Autodesk Fusion 360 part; units mm, degrees
note: some values were not read from the file. Chosen so that the rebuilt part matches the saved one: which bodies a step acts on; which face or edge a step refers to. Set by a fixed rule: which sketch regions a step uses.
(part 2 of 2)
sketch "Sketch2 (7)" plane through (0, 0, 0) normal (0.707107, 0, -0.707107) x (-0.707107, 0, -0.707107) in component "left (1) (1)"
  line L0 (273.05, 19.05) -> (228.6, 19.05)
  line L1 (228.6, 19.05) -> (228.6, 0)
  line L2 (228.6, 0) -> (273.05, 0)
  line L3 (273.05, 0) -> (273.05, 19.05)
  line L4 (234.95, 12.7) -> (266.7, 12.7)
  line L5 (266.7, 12.7) -> (266.7, 6.35)
  line L6 (266.7, 6.35) -> (234.95, 6.35)
  line L7 (234.95, 6.35) -> (234.95, 12.7)
  line L8 (243.84, 12.7) -> (243.84, 19.05) construction
  line L9 (261.9443, 6.35) -> (261.9443, 0) construction
  line L10 (266.7, 9.6711) -> (273.05, 9.6711) construction
  line L11 (234.95, 7.62) -> (228.6, 7.62) construction
  dimension "d230_1" = 6.35
  dimension "d231_1" = 6.35
  constraint horizontal L4
  constraint vertical L5
  constraint horizontal L6
  constraint vertical L7
  constraint coincident L4 L8.start
  constraint coincident L0 L8.end
  constraint perpendicular L0 L8
  constraint coincident L6 L9.start
  constraint perpendicular L6 L9
  constraint coincident L5 L10.start
  constraint coincident L3 L10.end
  constraint perpendicular L3 L10
  constraint coincident L7 L11.start
  constraint coincident L1 L11.end
  constraint perpendicular L1 L11
  constraint equal L10 L11
  constraint equal L8 L9
  constraint coincident L2 L9.end
  measures "d230_1" distance of L11.start L11.end
  measures "d231_1" distance of L8.start L8.end
extrude "Extrude2''''''''" cut sketch "Sketch2 (7)" against normal blind 12.7 contours L4 L5 L6 L7 bodies 23 in component "left (1) (1)"
sketch "Sketch1 (15)" plane through (0, 0, 0) normal (0.707107, 0, 0.707107) x (0.707107, 0, -0.707107) in component "front (1) (1)"
  line L0 (273.05, 0) -> (273.05, 19.05)
  line L1 (273.05, 19.05) -> (228.6, 19.05)
  line L2 (228.6, 19.05) -> (228.6, 0)
  line L3 (228.6, 0) -> (273.05, 0)
  line L4 (234.95, 12.7) -> (266.7, 12.7)
  line L5 (266.7, 12.7) -> (266.7, 6.35)
  line L6 (266.7, 6.35) -> (234.95, 6.35)
  line L7 (234.95, 6.35) -> (234.95, 12.7)
  line L8 (234.95, 11.43) -> (228.6, 11.43) construction
  line L9 (241.3, 12.7) -> (241.3, 19.05) construction
  line L10 (245.7528, 6.35) -> (245.7528, 0) construction
  line L11 (266.7, 9.525) -> (273.05, 9.525) construction
  dimension "d234_1" = 6.35
  dimension "d235_1" = 6.35
  dimension "d242_1" = 6.35
  dimension "d243_1" = 31.75
  constraint horizontal L4
  constraint vertical L5
  constraint horizontal L6
  constraint vertical L7
  constraint coincident L7 L8.start
  constraint coincident L2 L8.end
  constraint perpendicular L2 L8
  constraint coincident L4 L9.start
  constraint coincident L1 L9.end
  constraint perpendicular L1 L9
  constraint coincident L6 L10.start
  constraint coincident L3 L10.end
  constraint perpendicular L3 L10
  constraint coincident L5 L11.start
  constraint perpendicular L5 L11
  constraint equal L9 L10
  constraint equal L8 L11
  constraint midpoint L0 L11.end
  measures "d234_1" distance of L11.start L11.end
  measures "d235_1" distance of L10.start L10.end
  measures "d242_1" distance of L4.start L6.end
  measures "d243_1" distance of L4.start L4.end
extrude "Extrude1''''''''''''''" cut sketch "Sketch1 (15)" against normal blind 12.7 contours L4 L5 L6 L7 bodies 21 in component "front (1) (1)"
sketch "Sketch2 (8)" plane through (0, 0, 0) normal (-0.707107, 0, 0.707107) x (0.707107, 0, 0.707107) in component "front (1) (1)"
  line L0 (-228.6, 19.05) -> (-273.05, 19.05)
  line L1 (-273.05, 19.05) -> (-273.05, 0)
  line L2 (-273.05, 0) -> (-228.6, 0)
  line L3 (-228.6, 0) -> (-228.6, 19.05)
  line L4 (-266.7, 12.7) -> (-234.95, 12.7)
  line L5 (-234.95, 12.7) -> (-234.95, 6.35)
  line L6 (-234.95, 6.35) -> (-266.7, 6.35)
  line L7 (-266.7, 6.35) -> (-266.7, 12.7)
  line L8 (-241.3, 12.7) -> (-241.3, 19.05) construction
  line L9 (-234.95, 10.16) -> (-228.6, 10.16) construction
  line L10 (-266.7, 9.525) -> (-273.05, 9.525) construction
  line L11 (-256.54, 6.35) -> (-256.54, 0) construction
  dimension "d238_1" = 6.35
  dimension "d239_1" = 6.35
  dimension "d244_1" = 6.35
  dimension "d245_1" = 31.75
  constraint horizontal L4
  constraint vertical L5
  constraint horizontal L6
  constraint vertical L7
  constraint coincident L4 L8.start
  constraint coincident L0 L8.end
  constraint perpendicular L0 L8
  constraint coincident L5 L9.start
  constraint coincident L3 L9.end
  constraint perpendicular L3 L9
  constraint midpoint L7 L10.start
  constraint coincident L1 L10.end
  constraint perpendicular L1 L10
  constraint coincident L6 L11.start
  constraint coincident L2 L11.end
  constraint perpendicular L2 L11
  constraint equal L8 L11
  constraint equal L9 L10
  measures "d238_1" distance of L10.start L10.end
  measures "d239_1" distance of L11.start L11.end
  measures "d244_1" distance of L4.end L5.end
  measures "d245_1" distance of L5.end L6.end
extrude "Extrude2'''''''''" cut sketch "Sketch2 (8)" against normal blind 12.7 contours L4 L5 L6 L7 bodies 21 in component "front (1) (1)"
sketch "Sketch1 (16)" plane through (0, 6.35, 0) normal (0, 1, 0) x (-1, 0, 0) in component "LargeConnector (1)"
  line L0 (-207.5446, 207.5446) -> (-166.1347, 166.1347)
  line L1 (-166.1347, 166.1347) -> (-157.1545, 175.115)
  line L2 (-157.1545, 175.115) -> (-198.5644, 216.5249)
  line L3 (-198.5644, 216.5249) -> (-207.5446, 207.5446)
  line L4 (-219.9225, 194.7967) -> (-178.7929, 153.6671)
  line L5 (-178.7929, 153.6671) -> (-196.3942, 136.0658)
  line L6 (-196.3942, 136.0658) -> (-237.5238, 177.1954)
  line L7 (-237.5238, 177.1954) -> (-219.9225, 194.7967)
  dimension "d267_1" = 12.7
  dimension "d268_1" = 12.7
  dimension "d269_1" = 58.5624
  dimension "d270_1" = 58.166
  dimension "d271_1" = 24.892
  constraint parallel L1 L5
  constraint parallel L3 L7
  constraint parallel L0 L6
  constraint parallel L2 L4
  measures "d267_1" distance of L0.start L2.end
  measures "d268_1" distance of L0.end L1.end
  measures "d269_1" distance of L1.end L2.end
  measures "d270_1" distance of L4.start L4.end
  measures "d271_1" distance of L4.end L5.end
extrude "Extrude1'''''''''''''''" add sketch "Sketch1 (16)" along normal blind 5.842 separate body contours L4 L5 L6 L7 makes body 28 in component "LargeConnector (1)"
fillet "Fillet1''" radius 1.27 1 edges at (237.5238, 9.271, 177.1954) on bodies 28 in component "LargeConnector (1)"
fillet "Fillet2''" radius 1.27 3 edges at (228.2741, 12.192, 186.4451) (236.9977, 12.192, 177.1954) (216.51, 12.192, 156.1816) on bodies 28 in component "LargeConnector (1)"
fillet "Fillet3''" radius 1.27 3 edges at (216.51, 6.35, 156.1816) (236.9977, 6.35, 177.1954) (228.2741, 6.35, 186.4451) on bodies 28 in component "LargeConnector (1)"
fillet "Fillet4''" radius 1.27 5 edges at (198.9087, 12.192, 173.7829) (219.6595, 11.82, 194.5337) (219.9225, 9.271, 194.7967) (219.6595, 6.722, 194.5337) (198.9087, 6.35, 173.7829) on bodies 28 in component "LargeConnector (1)"
fillet "Fillet5''" radius 1.27 8 edges at (196.3942, 9.271, 136.0658) (196.1312, 11.82, 136.3289) (187.5936, 12.192, 144.8665) (179.0559, 11.82, 153.4041) (178.7929, 9.271, 153.6671) (179.0559, 6.722, 153.4041) (187.5936, 6.35, 144.8665) (196.1312, 6.722, 136.3289) on bodies 28 in component "LargeConnector (1)"
fillet "Fillet1'''" radius 1.27 1 edges at (-12.7, 9.2075, 266.192) on bodies 27 in component "Connector (1)"
fillet "Fillet2'''" radius 1.27 1 edges at (-12.7, 9.2075, 234.95) on bodies 27 in component "Connector (1)"
fillet "Fillet3'''" radius 1.27 5 edges at (0.381, 12.065, 234.95) (-12.328, 12.065, 235.322) (-12.7, 12.065, 250.571) (-12.328, 12.065, 265.82) (0.381, 12.065, 266.192) on bodies 27 in component "Connector (1)"
fillet "Fillet4'''" radius 1.27 5 edges at (12.192, 8.5725, 266.192) (12.192, 11.693, 265.82) (12.192, 12.065, 250.571) (12.192, 11.693, 235.322) (12.192, 8.5725, 234.95) on bodies 27 in component "Connector (1)"
fillet "Fillet5'''" radius 1.27 8 edges at (-0.254, 6.35, 266.192) (11.82, 6.35, 265.82) (12.192, 6.35, 250.571) (11.82, 6.35, 235.322) (-0.254, 6.35, 234.95) (-12.328, 6.35, 235.322) (-12.7, 6.35, 250.571) (-12.328, 6.35, 265.82) on bodies 27 in component "Connector (1)"
sketch "Sketch1 (17)" plane through (-85.1851, 123.3573, -56.3453) normal (0, 1, 0) x (-1, 0, 0) in component "Support"
  circle A0 centre (-261.1545, 121.8344) radius 12.7
  circle A1 centre (-261.458, -73.6679) radius 3.302
  circle A2 centre (-260.4003, 144.0466) radius 3.302
  circle A3 centre (-217.008, -150.6575) radius 3.302
  line L0 (-187.0949, 172.9094) -> (-237.485, 223.2995)
  arc A4 (-237.485, 223.2995) -> (-298.5003, 176.2263) centre (-25.4503, -114.6148) ccw
  line L1 (-298.5003, 176.2263) -> (-298.5003, 11.2648)
  arc A5 (-298.5003, 11.2648) -> (-218.5258, -181.8107) centre (-25.4503, 11.2648) ccw
  line L2 (-218.5258, -181.8107) -> (-187.0949, -150.3798)
  arc A6 (-187.0949, 172.9094) -> (-187.0949, -150.3798) centre (-25.4503, 11.2648) ccw
  arc A7 (-257.538, -54.7728) -> (-198.6844, -156.7103) centre (-25.4503, 11.2648) ccw
  arc A8 (-275.8608, -59.9863) -> (-212.3608, -169.9715) centre (-25.4503, 11.2648) ccw
  line L3 (-198.6844, -156.7103) -> (-212.3608, -169.9715)
  line L4 (-257.538, -54.7728) -> (-275.8608, -59.9863)
  line L5 (-25.4503, 11.2648) -> (-198.6844, -156.7103) construction
  line L6 (-198.6844, -156.7103) -> (-212.3608, -169.9715)
  line L7 (-25.4503, 11.2648) -> (-257.538, -54.7728) construction
  line L8 (-257.538, -54.7728) -> (-275.8608, -59.9863)
  line L9 (-261.458, -73.6679) -> (-257.538, -54.7728) construction
  line L10 (-261.458, -73.6679) -> (-275.8608, -59.9863) construction
  line L11 (-217.008, -150.6575) -> (-198.6844, -156.7103) construction
  line L12 (-217.008, -150.6575) -> (-212.3608, -169.9715) construction
  dimension "d344" = 241.3
  dimension "d345" = 19.05
  dimension "d346" = 127
  dimension "d351" = 6.604
  dimension "d352" = 6.604
  constraint coincident A5.centre A6.centre
  constraint collinear L5 L6
  constraint collinear L4 L7
  constraint coincident A1.centre L9.start
  constraint coincident A3.centre L11.start
  constraint equal L10 L12
  measures "d344" distance of A7.end A5.centre
  measures "d345" distance of A7.end A8.end
  measures "d346" distance of A8.start A8.end
  measures "d351" diameter of A3
  measures "d352" diameter of A1
extrude "Extrude1''''''''''''''''" add sketch "Sketch1 (17)" along normal blind 152.4 separate body contours A7 A8 L3 L4 L6 L8 makes body 29 in component "Support"
sketch "Sketch1 (18)" plane through (-85.1851, 123.3573, -56.3453) normal (0, 1, 0) x (-1, 0, 0) in component "eye"
  circle A0 centre (-261.1545, 121.8344) radius 12.7
  circle A1 centre (-261.458, -73.6679) radius 3.302
  circle A2 centre (-260.4003, 144.0466) radius 3.302
  circle A3 centre (-217.008, -150.6575) radius 3.302
  line L0 (-187.0949, 172.9094) -> (-237.485, 223.2995)
  arc A4 (-237.485, 223.2995) -> (-298.5003, 176.2263) centre (-25.4503, -114.6148) ccw
  line L1 (-298.5003, 176.2263) -> (-298.5003, 11.2648)
  arc A5 (-298.5003, 11.2648) -> (-218.5258, -181.8107) centre (-25.4503, 11.2648) ccw
  line L2 (-218.5258, -181.8107) -> (-187.0949, -150.3798)
  arc A6 (-187.0949, 172.9094) -> (-187.0949, -150.3798) centre (-25.4503, 11.2648) ccw
  arc A7 (-257.538, -54.7728) -> (-198.6844, -156.7103) centre (-25.4503, 11.2648) ccw
  line L3 (-198.6844, -156.7103) -> (-212.3608, -169.9715)
  line L4 (-257.538, -54.7728) -> (-275.8608, -59.9863)
  line L5 (-25.4503, 11.2648) -> (-198.6844, -156.7103) construction
  line L6 (-198.6844, -156.7103) -> (-212.3608, -169.9715)
  line L7 (-25.4503, 11.2648) -> (-257.538, -54.7728) construction
  line L8 (-257.538, -54.7728) -> (-275.8608, -59.9863)
  line L9 (-261.458, -73.6679) -> (-257.538, -54.7728) construction
  line L10 (-261.458, -73.6679) -> (-275.8608, -59.9863) construction
  line L11 (-217.008, -150.6575) -> (-198.6844, -156.7103) construction
  line L12 (-217.008, -150.6575) -> (-212.3608, -169.9715) construction
  line L13 (-212.3608, -169.9715) -> (-275.8608, -59.9863)
  dimension "d344_1" = 241.3
  dimension "d345_1" = 19.05
  dimension "d346_1" = 127
  dimension "d351_1" = 6.604
  dimension "d352_1" = 6.604
  constraint coincident A5.centre A6.centre
  constraint collinear L5 L6
  constraint collinear L4 L7
  constraint coincident A1.centre L9.start
  constraint coincident A3.centre L11.start
  constraint equal L10 L12
  measures "d344_1" distance of A7.end A5.centre
  measures "d345_1" distance of A7.end L3.end
  measures "d346_1" distance of L4.end L3.end
  measures "d351_1" diameter of A3
  measures "d352_1" diameter of A1
extrude "Extrude3" add sketch "Sketch1 (18)" along normal blind 88.9 separate body contours A7 L3 L4 L6 L8 L13 makes body 30 in component "eye"
sketch "Sketch2 (9)" plane through (193.3798, 0, -111.6479) normal (0.866025, 0, -0.5) x (-0.5, 0, -0.866025) in component "eye"
  line L0 (5.4083, 123.3573) -> (132.4083, 123.3573)
  line L1 (132.4083, 123.3573) -> (132.4083, 212.2573)
  line L2 (132.4083, 212.2573) -> (5.4083, 212.2573)
  line L3 (5.4083, 212.2573) -> (5.4083, 123.3573)
  line L4 (68.9083, 212.2573) -> (68.9083, 123.3573) construction
  line L5 (132.4083, 167.8073) -> (5.4083, 167.8073) construction
  circle A0 centre (68.9083, 167.8073) radius 34.925
  line L6 (33.9833, 202.7323) -> (103.8333, 202.7323) construction
  line L7 (103.8333, 202.7323) -> (103.8333, 132.8823) construction
  line L8 (103.8333, 132.8823) -> (33.9833, 132.8823) construction
  line L9 (33.9833, 132.8823) -> (33.9833, 202.7323) construction
  circle A1 centre (103.8333, 202.7323) radius 2.413
  circle A2 centre (103.8333, 132.8823) radius 2.413
  circle A3 centre (33.9833, 132.8823) radius 2.413
  circle A4 centre (33.9833, 202.7323) radius 2.413
  dimension "d357" = 69.85
  dimension "d358" = 4.826
  dimension "d359" = 4.826
  dimension "d360" = 4.826
  dimension "d361" = 4.826
  constraint midpoint L2 L4.start
  constraint midpoint L0 L4.end
  constraint midpoint L1 L5.start
  constraint midpoint L3 L5.end
  constraint midpoint L4 A0.centre
  constraint horizontal L6
  constraint vertical L7
  constraint horizontal L8
  constraint vertical L9
  constraint coincident L6.end L7.start
  constraint coincident L7 L8.start
  constraint coincident L7.end L8.start
  constraint coincident L8.end L9.start
  constraint coincident L6.start L9.end
  constraint tangent A0 L6
  constraint tangent A0 L9
  constraint tangent A0 L7
  constraint tangent A0 L8
  measures "d357" diameter of A0
  measures "d358" diameter of A1
  measures "d359" diameter of A2
  measures "d360" diameter of A3
  measures "d361" diameter of A4
extrude "Extrude4''" cut sketch "Sketch2 (9)" against normal blind 25.4 contours A0 bodies 30 in component "eye"
extrude "Extrude5" cut sketch "Sketch2 (9)" against normal blind 25.4 contours A1 | A2 | A3 | A4 bodies 30 in component "eye"
sketch "Sketch1 (19)" plane through (0, 123.3573, 0) normal (0, 1, 0) x (-1, 0, 0) in component "mirror"
  circle A0 centre (59.4654, -305.1611) radius 3.302
  line L0 (252.5409, -237.8866) -> (221.11, -206.4557)
  arc A1 (-102.1792, -206.4557) -> (221.11, -206.4557) centre (59.4654, -44.8111) ccw
  line L1 (-102.1792, -206.4557) -> (-133.6101, -237.8866)
  arc A2 (-133.6101, -237.8866) -> (-66.8314, -286.8967) centre (59.4654, -44.8111) ccw
  line L2 (-66.8314, -286.8967) -> (59.4654, -352.7861)
  line L3 (59.4654, -352.7861) -> (185.7622, -286.8967)
  arc A3 (185.7622, -286.8967) -> (252.5409, -237.8866) centre (59.4654, -44.8111) ccw
  circle A4 centre (59.4654, -44.8111) radius 45.2437
  circle A5 centre (59.4654, -44.8111) radius 46.0375
  dimension "d366" = 90.4875
  dimension "d367" = 92.075
  constraint concentric A1 A4
  constraint concentric A1 A5
  measures "d366" diameter of A4
  measures "d367" diameter of A5
extrude "Extrude1'''''''''''''''''" add sketch "Sketch1 (19)" along normal blind 106.68 separate body contours A5 makes body 31 in component "mirror"
sketch "Sketch2 (10)" plane through (0, 230.0373, 0) normal (0, 1, 0) x (-1, 0, 0) in component "mirror"
  circle A0 centre (59.4654, -44.8111) radius 46.0375
  circle A1 centre (59.4654, -44.8111) radius 46.0375
  circle A2 centre (59.4654, -44.8111) radius 45.2438
extrude "Extrude2''''''''''" add sketch "Sketch2 (10)" along normal blind 6.35 separate body contours A0 A1 | A2 makes body 32 in component "mirror"
sketch "Sketch3 (3)" plane through (0, 236.3873, 0) normal (0, 1, 0) x (-1, 0, 0) in component "mirror"
  circle A0 centre (59.4654, -44.8111) radius 46.0375
  circle A1 centre (59.4654, -44.8111) radius 28.575
  dimension "d372" = 57.15
  constraint concentric A0 A1
  measures "d372" diameter of A1
extrude "Extrude3'" add sketch "Sketch3 (3)" along normal blind 6.35 and the other way blind 101.6 contours A1 bodies 32 in component "mirror"
sketch "Sketch4" plane through (0, 0, 0) normal (0, 0, 1) x (1, 0, 0) in component "mirror"
  line L0 (-105.5029, 133.0613) -> (-16.3489, 133.0613) construction
  line L1 (-105.5029, 230.0373) -> (-105.5029, 217.3373) construction
  line L2 (-105.5029, 217.3373) -> (-16.3489, 133.0613)
  line L3 (-105.5029, 217.3373) -> (-105.5029, 133.0613) construction
  line L4 (-16.3489, 133.0613) -> (-16.3489, 145.7613) construction
  line L5 (-105.5029, 230.0373) -> (-16.3489, 145.7613) construction
  line L6 (-105.5029, 217.3373) -> (-121.6701, 232.6199)
  line L7 (-121.6701, 232.6199) -> (-121.6701, 245.3199) construction
  line L8 (-121.6701, 245.3199) -> (-105.5029, 230.0373) construction
  line L9 (-16.3489, 145.7613) -> (-0.1433, 130.4425) construction
  line L10 (-0.1433, 130.4425) -> (-0.1433, 117.7425)
  line L11 (-0.1433, 117.7425) -> (-16.3489, 133.0613)
  line L12 (-121.6701, 232.6199) -> (-121.6701, 119.38)
  line L13 (-121.6701, 119.38) -> (-0.1433, 117.7425)
  dimension "d377" = 12.7
  dimension "d379" = 122.682
  dimension "d380" = 89.154
  dimension "d381" = 84.276
  dimension "d382" = 12.7
  constraint horizontal L0
  constraint vertical L1
  constraint perpendicular L0 L3
  constraint perpendicular L0 L4
  constraint parallel L2 L6
  constraint parallel L1 L7
  constraint parallel L5 L9
  constraint parallel L4 L10
  constraint collinear L2 L11
  constraint collinear L5 L8
  constraint parallel L7 L12
  measures "d377" distance of L1.start L1.end
  measures "d379" distance of L0.end L1.end
  measures "d380" distance of L0.start L0.end
  measures "d381" distance of L0.start L1.end
  measures "d382" distance of L0.end L4.end
extrude "Extrude4'''" cut sketch "Sketch4" along normal mid plane 254 bodies 31 in component "mirror"
extrude "Extrude5'" cut sketch "Sketch4" against normal blind 101.6 bodies 32 in component "mirror"
sketch "Sketch5" plane through (0, 0, 0) normal (0, 0, 1) x (1, 0, 0) in component "mirror"
  line L0 (-121.6701, 245.3199) -> (-0.1433, 130.4425)
  line L1 (-121.6701, 245.3199) -> (-121.6701, 133.4962)
  line L2 (-121.6701, 133.4962) -> (-0.1433, 130.4425)
  point P0 (-121.6701, 245.3199)
  point P1 (-0.1433, 130.4425)
  constraint coincident P0 L0.start
  constraint coincident P1 L0.end
  constraint vertical L1
extrude "Extrude6" cut sketch "Sketch5" against normal blind 101.6 bodies 32 in component "mirror"
hole "Hole1" at (-59.4654, 242.7373, -45.1004) direction (0, -1, 0) diameter 4.826 depth 127 tip angle 180 bodies 32 in component "mirror"
sketch "Sketch6" plane through (0, 0, 0) normal (0, 1, 0) x (1, 0, 0) in component "mirror"
  circle A0 centre (-59.4654, 45.1004) radius 9.525
  circle A1 centre (-59.4654, 45.1004) radius 2.413
  dimension "d392" = 19.05
  constraint concentric A0 A1
  measures "d392" diameter of A0
extrude "Extrude7" cut sketch "Sketch6" along normal blind 233.68 bodies 32 in component "mirror"
combine "Combine1" operation add target body 32 tool bodies 31 in component "mirror"
component "Top Plate" placed x (1, 0, 0) y (0, 1, 0) z (0, 0, 1) at (-58.8676, 104.3073, -45.4397)
component "Slice1" placed x (0.707107, 0, 0.707107) y (0, 1, 0) z (-0.707107, 0, 0.707107) at (0, 0, 0)
component "Slice2" placed x (0.707107, 0, -0.707107) y (0, 1, 0) z (0.707107, 0, 0.707107) at (0, 0, 0)
component "Bottom Plate" placed x (1, 0, 0) y (0, 1, 0) z (0, 0, 1) at (-58.8676, 104.3073, -45.4397)
component "Support" placed x (1, 0, 0) y (0, 1, 0) z (0, 0, 1) at (0, 0, 0)
component "Support" placed x (1, 0, 0) y (0, 1, 0) z (0, 0, 1) at (0, 0, 0)
component "Support" placed x (1, 0, 0) y (0, 1, 0) z (0, 0, 1) at (0, 0, 0)
component "Support" placed x (1, 0, 0) y (0, 1, 0) z (0, 0, 1) at (0, 0, 0)
component "eye" placed x (1, 0, 0) y (0, 1, 0) z (0, 0, 1) at (0, 0, 0)
component "mirror" placed x (1, 0, 0) y (0, 1, 0) z (0, 0, 1) at (0, 0, 0)
component "right (1)" placed x (1, 0, 0) y (0, 1, 0) z (0, 0, 1) at (-0.8672, 0, 0.3592) in component "Top Plate"
component "front (1)" placed x (1, 0, 0) y (0, 1, 0) z (0, 0, 1) at (-0.5978, 0, 0.6286) in component "Top Plate"
component "rear (1)" placed x (1, 0, 0) y (0, 1, 0) z (0, 0, 1) at (0, 0, 0) in component "Top Plate"
component "left (1)" placed x (1, 0, 0) y (0, 1, 0) z (0, 0, 1) at (-0.2386, 0, 0.2694) in component "Top Plate"
component "Connector" placed x (0.707107, 0, 0.707107) y (0, 1, 0) z (-0.707107, 0, 0.707107) at (354.6303, 0.3175, -354.4507) in component "front (1)"
component "Connector" placed x (0.707107, 0, -0.707107) y (0, 1, 0) z (0.707107, 0, 0.707107) at (-354.1813, 0.3175, -354.8997) in component "front (1)"
component "Connector" placed x (1, 0, 0) y (0, 1, 0) z (0, 0, 1) at (0, 0.3175, 0.254) in component "rear (1)"
component "left (2)" placed x (1, 0, 0) y (0, 1, 0) z (0, 0, 1) at (0, 0, 0) in component "rear (1)"
component "right (2)" placed x (1, 0, 0) y (0, 1, 0) z (0, 0, 1) at (-0.508, 0, 0) in component "rear (1)"
component "LargeConnector" placed x (0, 0, -1) y (0, 1, 0) z (1, 0, 0) at (-352.6891, 0.254, 395.0878) in component "rear (1)"
component "LargeConnector" placed x (1, 0, 0) y (0, 1, 0) z (0, 0, 1) at (-22.0063, 0.254, 21.588) in component "rear (1)"
component "right (1) (1)" placed x (1, 0, 0) y (0, 1, 0) z (0, 0, 1) at (-0.8672, 0, 0.3592) in component "Bottom Plate"
component "front (1) (1)" placed x (1, 0, 0) y (0, 1, 0) z (0, 0, 1) at (-0.5978, 0, 0.6286) in component "Bottom Plate"
component "rear (1) (1)" placed x (1, 0, 0) y (0, 1, 0) z (0, 0, 1) at (0, 0, 0) in component "Bottom Plate"
component "left (1) (1)" placed x (1, 0, 0) y (0, 1, 0) z (0, 0, 1) at (-0.2386, 0, 0.2694) in component "Bottom Plate"
component "Connector (1)" placed x (0.707107, 0, 0.707107) y (0, 1, 0) z (-0.707107, 0, 0.707107) at (354.6303, 0.3175, -354.4507) in component "front (1) (1)"
component "Connector (1)" placed x (0.707107, 0, -0.707107) y (0, 1, 0) z (0.707107, 0, 0.707107) at (-354.1813, 0.3175, -354.8997) in component "front (1) (1)"
component "Connector (1)" placed x (1, 0, 0) y (0, 1, 0) z (0, 0, 1) at (0, 0.3175, 0.254) in component "rear (1) (1)"
component "left (2) (1)" placed x (1, 0, 0) y (0, 1, 0) z (0, 0, 1) at (0, 0, 0) in component "rear (1) (1)"
component "right (2) (1)" placed x (1, 0, 0) y (0, 1, 0) z (0, 0, 1) at (-0.508, 0, 0) in component "rear (1) (1)"
component "LargeConnector (1)" placed x (0, 0, -1) y (0, 1, 0) z (1, 0, 0) at (-352.6891, 0.254, 395.0878) in component "rear (1) (1)"
component "LargeConnector (1)" placed x (1, 0, 0) y (0, 1, 0) z (0, 0, 1) at (-22.0063, 0.254, 21.588) in component "rear (1) (1)"
equation "d22_2 = 3 1/8\""
equation "d162_1 = d350"
equation "d163_1 = d350"
equation "d167_1 = 1 3/4\""
equation "d172_1 = d350"
equation "d174_1 = d350"
equation "d176_1 = d350"
equation "d177_1 = d350"
equation "d179_1 = d350"
equation "d180_1 = d350"
equation "d22_2_1 = 3 1/8\""
equation "d162_1_1 = d350"
equation "d163_1_1 = d350"
equation "d167_1_1 = 1 3/4\""
equation "d172_1_1 = d350"
equation "d174_1_1 = d350"
equation "d176_1_1 = d350"
equation "d177_1_1 = d350"
equation "d179_1_1 = d350"
equation "d180_1_1 = d350"
equation "d349 = d350"
equation "d366 = 3 9/16\""
equation "d367 = d366 + ( 1 / 16 ) * 1 in"
